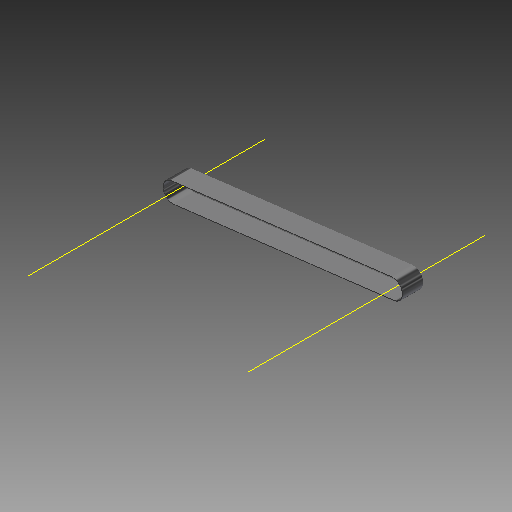
# Autodesk Inventor part: Synchronous Belt
Saved by Autodesk Inventor 2019.4 (Build 234330000, 330)
## iProperties
Created: 2020-01-11
Part Number: Synchronous Belt
Material: Rubber
Document SubType Name: Modeling
Designer: admin
Density: 0.93 g/cm^3
Appearance: Rubber - Black - Version 1.1
Mass: 14.415 g
Surface Area: 322.4 cm^2
Volume: 15.5 cm^3
CustomPartVersion: 1
Author: admin
Autodesk Inventor part; units mm, degrees
ref_plane "YZ Plane" through (0, 0, 0) normal (1, 0, 0) x (0, 1, 0)
ref_plane "XZ Plane" through (0, 0, 0) normal (0, 1, 0) x (-1, 0, 0)
ref_plane "XY Plane" through (0, 0, 0) normal (0, 0, 1) x (1, 0, 0)
sketch "Sketch Path" plane through (0, 0, 0) normal (0, 0, 1) x (1, 0, 0)
  arc A0 (-86.9778, -25.6677) -> (-89.8604, -1.9691) centre (-88.4191, -13.8184) ccw
  arc A1 (-360.3666, -34.8733) -> (-357.4839, -58.5718) centre (-358.9252, -46.7226) ccw
  line L0 (-360.3666, -34.8733) -> (-89.8604, -1.9691)
  line L1 (-86.9778, -25.6677) -> (-357.4839, -58.5718)
  constraints: 4 end point, 4 point on circle, 2 centre point
ref_plane "Cross Section Plane" through (-89.8604, -1.9691, 0) normal (-0.992683, -0.1207492, 0) x (0, 0, 1)
ref_plane "Work Plane2" through (-88.4191, -13.8184, 0) normal (-1, 0, 0) x (0, 0, 1)
ref_plane "Work Plane3" through (-358.9252, -46.7226, 0) normal (1, 0, 0) x (0, 0, 1)
sketch "Cross Section" plane through (-89.8604, -1.9691, 0) normal (-0.992683, -0.1207492, 0) x (0, 0, 1)
  line L0 (-12.5, 0.5) -> (12.5, 0.5)
  line L1 (12.5, 0.5) -> (12.5, -0.5)
  line L2 (12.5, -0.5) -> (-12.5, -0.5)
  line L3 (-12.5, -0.5) -> (-12.5, 0.5)
  line L4 (-12.5, 0) -> (12.5, 0) construction
  point P0 (0, 0)
  point P1 (0, 0)
  dimension "d0" = 25
  dimension "d4" = 0.5
  dimension "d5" = 0.5
  constraints: 10 end point, 3 midpoint, 2 parallel, 1 coincident, 1 horizontal, 1 perpendicular, 1 other
  measures "d0" distance between parallel lines of L1 L3
  measures "d4" distance between parallel lines of L2 L4
  measures "d5" distance between parallel lines of L4 L0
sweep "Belt" add profiles "Cross Section" path "Sketch Path" path curves L1 A1 L0 A0
equation "\"d0\" = da_B"
equation "\"d4\" = da_a"
equation "\"d5\" = da_a2"
equation "\"da_B\" = 25"
equation "\"da_pb\" = 5"
equation "\"da_a\" = 0.5"
equation "\"da_S\" = 2.65"
equation "\"da_Beta\" = 20deg"
equation "\"da_Ht\" = 1.2"
equation "\"da_H\" = 2.2"
equation "\"da_a2\" = 0.5"
body "Solid1"
